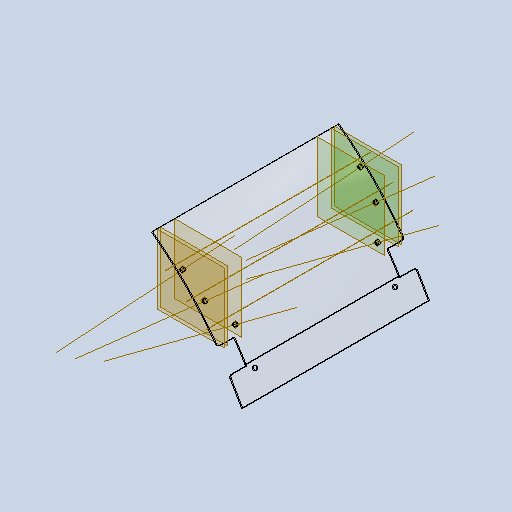
# Autodesk Inventor part: ! Intake polycarb
Saved by Autodesk Inventor 2023.2 (Build 272271030, 271C)
## iProperties
Created: 2023-05-27
Part Number: ! Intake polycarb
Material: Polycarbonate, Clear
Document SubType Name: Modeling
Designer: Main Account
Density: 1.2 g/cm^3
Appearance: Polycarbonate - Clear
Author: Main Account
Autodesk Inventor part; units mm, degrees
ref_plane "YZ Plane" through (0, 0, 0) normal (1, 0, 0) x (0, 1, 0)
ref_plane "XZ Plane" through (0, 0, 0) normal (0, 1, 0) x (-1, 0, 0)
ref_plane "XY Plane" through (0, 0, 0) normal (0, 0, 1) x (1, 0, 0)
sketch "Sketch1" plane through (0, 0, 0) normal (0, 0, 1) x (1, 0, 0)
  line L0 (17.2421, 103.0289) -> (10.8921, 114.0275) projected
  arc A0 (-38.1, 178.1746) -> (-35.7188, 175.7934) centre (-35.7188, 178.1746) ccw construction
  line L1 (-57.8926, 195.9643) -> (-60.8346, 198.1519) construction
  line L2 (-54.5271, 197.4183) -> (-57.8926, 195.9643) construction
  line L3 (-60.8346, 198.1519) -> (-60.4111, 201.7935) construction
  circle A1 centre (-57.4691, 199.6059) radius 4.7625 construction
  line L4 (26.0216, 87.8223) -> (10.8921, 114.0275)
  arc A2 (10.8921, 114.0275) -> (-77.4031, 211.1891) centre (-275.2793, -57.3297) ccw
  line L5 (24.6468, 87.0285) -> (9.5236, 113.2227)
  arc A3 (9.5236, 113.2227) -> (-78.349, 209.9142) centre (-275.2793, -57.3297) ccw
  line L6 (26.0216, 87.8223) -> (24.6468, 87.0285)
  line L7 (-77.4031, 211.1891) -> (-78.349, 209.9142)
  arc A4 (8.2879, 112.4961) -> (-75.5859, 206.0593) centre (-275.2793, -57.3297) ccw construction
  line L8 (8.2879, 112.4961) -> (24.1221, 85.0704) construction
  point P0 (0, 0)
  dimension "d0" = 1.5875
  dimension "d26" = 1.4334
  constraints: 10 end point, 7 point on circle, 3 centre point, 1 perpendicular, 1 point on line, 1 tangent, 4 other
  measures "d0" distance between parallel lines of L4 L5
  measures "d26" distance between parallel lines of L5 L8
extrude "main extrusion" add sketch "Sketch1" against normal blind 213.36
sketch "Sketch2" plane through (9.5236, 113.2227, -213.36) normal (-0.866, -0.5, 0) x (0, 0, 1)
  line L0 (213.36, -30.2465) -> (213.36, 0.0127) projected
  line L1 (213.36, -1.1707) -> (194.31, -1.1707)
  line L2 (194.31, -1.1707) -> (194.31, 24.2293)
  line L3 (194.31, 24.2293) -> (213.36, 24.2293)
  line L4 (213.36, 24.2293) -> (213.36, -1.1707)
  line L5 (194.31, -1.1707) -> (0, -1.1707) construction
  line L6 (213.36, 0.0127) -> (0, 0.0127) construction
  line L7 (0, -1.1707) -> (19.05, -1.1707)
  line L8 (19.05, -1.1707) -> (19.05, 24.2293)
  line L9 (19.05, 24.2293) -> (0, 24.2293)
  line L10 (0, 24.2293) -> (0, -1.1707)
  point P0 (213.36, -93.292)
  dimension "d3" = 19.05
  dimension "d4" = 25.4
  dimension "d5" = 19.05
  dimension "d6" = 25.4
  constraints: 18 end point, 5 parallel, 3 horizontal, 2 perpendicular, 1 point on line, 1 vertical
  measures "d3" distance of L2.end L3.end
  measures "d4" distance of L1.end L2.end
  measures "d5" distance of L9.end L8.end
  measures "d6" distance of L8.end L7.end
extrude "square side cuts" cut sketch "Sketch2" along normal blind 2.54 and the other way blind 2.54
fillet "square cut fillets" radius 2.54 4 edges at (-3.004, 133.9675, -213.36) (-3.004, 133.9675, 0) (10.7964, 112.6057, 0) (10.7964, 112.6057, -213.36)
ref_plane "Work Plane1" through (0, 0, -5.08) normal (0, 0, 1) x (1, 0, 0)
ref_plane "Work Plane2" through (-50.8851, 191.5138, -213.36) normal (-0.8031, 0.5959, 0) x (0, 0, 1)
hole "Hole1" at (-48.3442, 184.9538, -5.08) direction (0.6836, 0.7298, 0) diameter 4.2418 depth 12.7
ref_plane "Work Plane3" through (0, 0, -8.89) normal (0, 0, 1) x (1, 0, 0)
ref_plane "Work Plane4" through (-26.407, 173.352, -213.36) normal (-0.8031, 0.5959, 0) x (0, 0, 1)
hole "Hole2" at (-26.8136, 162.8194, -8.89) direction (0.7485, 0.6632, 0) diameter 4.2418 depth 12.7
ref_plane "Work Plane5" through (0, 0, -25.4) normal (0, 0, 1) x (1, 0, 0)
ref_plane "Work Plane6" through (-3.9687, 156.7036, -213.36) normal (-0.8031, 0.5959, 0) x (0, 0, 1)
hole "Hole5" at (-8.6418, 140.4208, -25.4) direction (0.8032, 0.5957, 0) diameter 4.2418 depth 12.7
ref_plane "Work Plane7" through (0, 0, -208.28) normal (0, 0, -1) x (-1, 0, 0)
ref_plane "Work Plane8" through (-50.8851, 191.5138, -213.36) normal (-0.8031, 0.5959, 0) x (0, 0, 1)
hole "Hole6" at (-48.3442, 184.9538, -208.28) direction (0.6836, 0.7298, 0) diameter 4.2418 depth 12.7
ref_plane "Work Plane9" through (0, 0, -204.47) normal (0, 0, -1) x (-1, 0, 0)
ref_plane "Work Plane10" through (-26.407, 173.352, -213.36) normal (-0.8031, 0.5959, 0) x (0, 0, 1)
hole "Hole7" at (-26.8136, 162.8194, -204.47) direction (0.7485, 0.6632, 0) diameter 4.2418 depth 12.7
ref_plane "Work Plane11" through (0, 0, -187.96) normal (0, 0, -1) x (-1, 0, 0)
ref_plane "Work Plane12" through (-3.9687, 156.7036, -213.36) normal (-0.8031, 0.5959, 0) x (0, 0, 1)
hole "Hole8" at (-8.6418, 140.4208, -187.96) direction (0.8032, 0.5957, 0) diameter 4.2418 depth 12.7
sketch "Sketch4" plane through (24.6468, 87.0285, -213.36) normal (-0.866, -0.5, 0) x (0, 0, 1)
  circle A0 centre (26.67, 23.9091) radius 2.1209
  circle A1 centre (186.69, 23.9091) radius 2.1209
  arc A2 (22.0345, 23.9091) -> (26.2255, 23.9091) centre (24.13, 23.9091) ccw construction
  line L0 (24.13, 23.9091) -> (26.67, 23.9091) construction
  arc A3 (187.1345, 23.9091) -> (191.3255, 23.9091) centre (189.23, 23.9091) ccw construction
  line L1 (189.23, 23.9091) -> (186.69, 23.9091) construction
  point P0 (213.36, -63.0455)
  dimension "d102" = 4.2418
  dimension "d105" = 4.2418
  dimension "d109" = 2.54
  dimension "d110" = 2.54
  constraints: 4 end point, 2 centre point, 2 coincident, 2 horizontal, 1 other
  measures "d102" diameter of A0
  measures "d105" diameter of A1
  measures "d109" distance of L0.start L0.end
  measures "d110" distance of L1.start L1.end
extrude "top screw holes" cut sketch "Sketch4" against normal blind 1.5875
body "Solid1"
